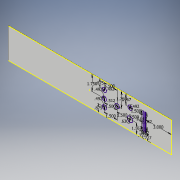
# Autodesk Inventor part: Faceplate
Saved by Autodesk Inventor 2017 (Build 210142000, 142)
## iProperties
Created: 2017-03-30
Part Number: Faceplate
Material: Generic
Document SubType Name: Modeling
Designer: plumbj
Density: 1 g/cm^3
Appearance: Default
Author: plumbj
Autodesk Inventor part; units mm, degrees
ref_plane "YZ Plane" through (0, 0, 0) normal (1, 0, 0) x (0, 1, 0)
ref_plane "XZ Plane" through (0, 0, 0) normal (0, 1, 0) x (-1, 0, 0)
ref_plane "XY Plane" through (0, 0, 0) normal (0, 0, 1) x (1, 0, 0)
sketch "Sketch1" plane through (0, 0, 0) normal (0, 0, 1) x (1, 0, 0)
  line L0 (-240.6762, -44.1472) -> (241.9238, -44.1472)
  line L1 (241.9238, -44.1472) -> (241.9238, 44.7528)
  line L2 (241.9238, 44.7528) -> (-240.6762, 44.7528)
  line L3 (-240.6762, 44.7528) -> (-240.6762, -44.1472)
  point P0 (0, 0)
  dimension "d0" = 482.6
  dimension "d1" = 88.9
  constraints: 8 end point, 2 parallel, 1 horizontal, 1 perpendicular
  measures "d0" distance of L2.end L1.end
  measures "d1" distance of L1.end L0.end
extrude "Extrusion1" add sketch "Sketch1" along normal blind 1.1113
sketch "Sketch2" plane through (0, 0, 1.1113) normal (0, 0, 1) x (1, 0, 0)
  point P0 (0, 0)
sketch "Sketch3" plane through (0, 0, 1.1113) normal (0, 0, 1) x (1, 0, 0)
  point P0 (0, 0)
sketch "Sketch4" plane through (0, 0, 1.1113) normal (0, 0, 1) x (1, 0, 0)
  line L0 (157.5238, 26.3059) -> (160.1238, 26.3059)
  line L1 (160.1238, 26.3059) -> (160.1238, -25.6941)
  line L2 (160.1238, -25.6941) -> (157.5238, -25.6941)
  line L3 (157.5238, -25.6941) -> (157.5238, 26.3059)
  line L4 (163.1238, 26.3059) -> (165.7238, 26.3059)
  line L5 (165.7238, 26.3059) -> (165.7238, -25.6941)
  line L6 (165.7238, -25.6941) -> (163.1238, -25.6941)
  line L7 (163.1238, -25.6941) -> (163.1238, 26.3059)
  line L8 (-240.6762, -44.1472) -> (241.9238, -44.1472) projected
  line L9 (241.9238, -44.1472) -> (241.9238, 44.7528) projected
  circle A0 centre (43.2238, -21.9222) radius 6.2484
  circle A1 centre (43.2238, 0.3028) radius 6.2484
  circle A2 centre (119.4238, 15.1195) radius 6.2484
  circle A3 centre (43.2238, 22.5278) radius 6.2484
  circle A4 centre (81.3238, 0.3028) radius 6.5
  circle A5 centre (119.4238, -14.5139) radius 8
  line L10 (241.9238, 44.7528) -> (-240.6762, 44.7528) projected
  point P0 (0, 0)
  dimension "d9" = 2.6
  dimension "d12" = 2.6
  dimension "d13" = 52
  dimension "d16" = 3
  dimension "d17" = 18.4531
  dimension "d18" = 52
  dimension "d20" = 18.4531
  dimension "d21" = 76.2
  dimension "d22" = 12.4968
  dimension "d23" = 12.4968
  dimension "d24" = 12.4968
  dimension "d25" = 12.4968
  dimension "d26" = 13
  dimension "d27" = 16
  dimension "d28" = 38.1
  dimension "d35" = 44.45
  dimension "d36" = 44.45
  dimension "d37" = 22.225
  dimension "d38" = 22.225
  dimension "d39" = 29.6333
  dimension "d40" = 29.6333
  dimension "d41" = 38.1
  dimension "d42" = 38.1
  dimension "d43" = 38.1
  dimension "d44" = 38.1
  dimension "d45" = 38.1
  constraints: 16 end point, 6 centre point, 4 parallel, 2 horizontal, 2 perpendicular
  measures "d9" distance of L1.end L2.end
  measures "d12" distance of L5.end L6.end
  measures "d13" distance of L4.end L5.end
  measures "d16" distance between parallel lines of L7 L1
  measures "d17" distance between parallel lines of L8 L2
  measures "d18" distance between parallel lines of L2 L0
  measures "d20" distance between parallel lines of L8 L6
  measures "d21" distance between parallel lines of L9 L5
  measures "d22" diameter of A0
  measures "d23" diameter of A1
  measures "d24" diameter of A2
  measures "d25" diameter of A3
  measures "d26" diameter of A4
  measures "d27" diameter of A5
  measures "d28" distance from line of L3 A5.centre
  measures "d35" distance from line of L10 A4.centre
  measures "d36" distance from line of L10 A1.centre
  measures "d37" distance from line of L10 A3.centre
  measures "d38" distance from line of L8 A0.centre
  measures "d39" distance from line of L10 A2.centre
  measures "d40" distance from line of L8 A5.centre
  measures "d41" distance from line of L3 A2.centre
  measures "d42" horizontal distance of A5.centre A4.centre
  measures "d43" distance of A4.centre A1.centre
  measures "d44" horizontal distance of A4.centre A3.centre
  measures "d45" horizontal distance of A0.centre A4.centre
sketch "Sketch5" plane through (0, 0, 1.1113) normal (0, 0, 1) x (1, 0, 0)
  point P0 (0, 0)
body "Solid1"
